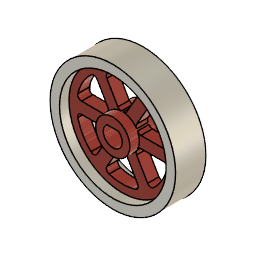
Flywheel (Autodesk Fusion 360 design; units mm, degrees)
Autodesk Fusion 360 part; units mm, degrees
sketch "Sketch1" plane through (0, 0, 0) normal (0, 1, 0) x (1, 0, 0)
  circle A0 centre (0, 0) radius 16.5
  dimension "d1" = 33
  constraint coincident A0.centre origin
  measures "d1" diameter of A0
extrude "Extrude1" add sketch "Sketch1" along normal blind 8
ref_plane "WorkPlane1" through (0, 4, 0) normal (0, -1, 0) x (-1, 0, 0)
sketch "Sketch2" plane through (0, 0, 0) normal (0, -1, 0) x (1, 0, 0)
  circle A0 centre (0, 0) radius 16.5
  circle A1 centre (0, 0) radius 14
  dimension "d4" = -2.5
extrude "Extrude2" cut sketch "Sketch2" against normal blind 2.5 contours A1
mirror "Mirror1" about plane through (0, 4, 0) normal (0, -1, 0) of "Extrude2"
hole "Hole3" at (0, 2.5, 0) direction (0, 1, 0) diameter 5 end through all
sketch "Sketch5" plane through (0, 2.5, 0) normal (0, -1, 0) x (1, 0, 0)
  circle A0 centre (0, 0) radius 2.5
  circle A1 centre (0, 0) radius 14
  circle A2 centre (0, 0) radius 4.5
  dimension "d22" = 2
extrude "Extrude4" add sketch "Sketch5" against normal up to surface (8 mm away) from surface at 2.5 contours A2
sketch "Sketch8" plane through (0, 2.5, 0) normal (0, -1, 0) x (1, 0, 0)
  circle A0 centre (0, 0) radius 4.5
  circle A1 centre (0, 0) radius 14
  circle A2 centre (0, 0) radius 12
  line L0 (-4.5, 0) -> (-12, 0)
  line L1 (-4.2426, 1.5) -> (-11.9059, 1.5)
  line L2 (-4.2426, -1.5) -> (-11.9059, -1.5)
  line L3 (-3.4204, -2.9242) -> (-7.252, -9.5608)
  line L4 (-0.8223, -4.4242) -> (-4.6539, -11.0608)
  line L5 (0.8223, -4.4242) -> (4.6539, -11.0608)
  line L6 (3.4204, -2.9242) -> (7.252, -9.5608)
  line L7 (4.2426, -1.5) -> (11.9059, -1.5)
  line L8 (4.2426, 1.5) -> (11.9059, 1.5)
  line L9 (3.4204, 2.9242) -> (7.252, 9.5608)
  line L10 (0.8223, 4.4242) -> (4.6539, 11.0608)
  line L11 (-0.8223, 4.4242) -> (-4.6539, 11.0608)
  line L12 (-3.4204, 2.9242) -> (-7.252, 9.5608)
  dimension "d30" = -2
  dimension "d31" = 1.5
  dimension "d33" = 360
  constraint coincident A0 L0.start
  constraint coincident A2 L0.end
  constraint horizontal L0
  constraint coincident A0 L1.start
  constraint coincident A2 L1.end
  constraint horizontal L1
  constraint symmetric L0 L1.start L2.start
  constraint symmetric L0 L1.end L2.end
  measures "d31" distance of L0 L1
extrude "Extrude6" cut sketch "Sketch8" against normal through all contours A0 A2 L8 L9 | A0 A2 L6 L7 | A0 A2 L10 L11 | A0 A2 L4 L5 | A0 A2 L1 L12 | A0 A2 L2 L3
fillet "Fillet1" radius 1 24 edges at (11.9059, 4, 1.5) (4.2426, 4, 1.5) (3.4204, 4, 2.9242) (7.252, 4, 9.5608) (4.6539, 4, 11.0608) (0.8223, 4, 4.4242) (-0.8223, 4, 4.4242) (-4.6539, 4, 11.0608) (4.2426, 4, -1.5) (3.4204, 4, -2.9242) (11.9059, 4, -1.5) (7.252, 4, -9.5608) (0.8223, 4, -4.4242) (-0.8223, 4, -4.4242) (-4.6539, 4, -11.0608) (4.6539, 4, -11.0608) (-7.252, 4, 9.5608) (-11.9059, 4, 1.5) (-3.4204, 4, 2.9242) (-4.2426, 4, 1.5) (-11.9059, 4, -1.5) (-7.252, 4, -9.5608) (-3.4204, 4, -2.9242) (-4.2426, 4, -1.5)
sketch "Sketch9" plane through (0, 0, 0) normal (0, -1, 0) x (1, 0, 0)
  circle A0 centre (0, 0) radius 2.5
  circle A1 centre (0, 0) radius 4.5
  line L0 (1.5, 2) -> (-1.5, 2)
  dimension "d37" = 2
  constraint coincident A0 L0.start
  constraint coincident A0 L0.end
  constraint horizontal L0
  measures "d37" distance of A0.centre L0
extrude "Extrude7" add sketch "Sketch9" against normal up to surface (8 mm away) contours A0 L0 picked at (-0.3999, 2.0645)
